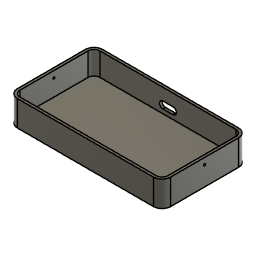
Case (INCOMPLETE) (Autodesk Fusion 360 design; units mm, degrees)
Autodesk Fusion 360 part; units mm, degrees
sketch "Sketch1" plane through (0, 0, 0) normal (0, 1, 0) x (1, 0, 0)
  line L0 (-80, 50) -> (80, 50)
  line L1 (90, 40) -> (90, -40)
  line L2 (80, -50) -> (-80, -50)
  line L3 (-90, -40) -> (-90, 40)
  line L4 (-90, 50) -> (90, -50) construction
  line L5 (90, 50) -> (-90, -50) construction
  arc A0 (-90, -40) -> (-80, -50) centre (-80, -40) ccw
  arc A1 (80, -50) -> (90, -40) centre (80, -40) ccw
  arc A2 (90, 40) -> (80, 50) centre (80, 40) ccw
  arc A3 (-80, 50) -> (-90, 40) centre (-80, 40) ccw
  arc A4 (87, 40) -> (80, 47) centre (80, 40) ccw
  line L6 (-80, 47) -> (80, 47)
  arc A5 (-80, 47) -> (-87, 40) centre (-80, 40) ccw
  line L7 (-87, -40) -> (-87, 40)
  arc A6 (-87, -40) -> (-80, -47) centre (-80, -40) ccw
  line L8 (80, -47) -> (-80, -47)
  arc A7 (80, -47) -> (87, -40) centre (80, -40) ccw
  line L9 (87, 40) -> (87, -40)
  dimension "d1" = 180
  dimension "d2" = 100
  dimension "d3" = 10
  dimension "d4" = 3
  constraint horizontal L0
  constraint perpendicular L0 L1
  constraint parallel L0 L2
  constraint parallel L1 L3
  constraint coincident L4 origin
  constraint coincident L5 origin
  constraint coincident L5.end L3
  constraint coincident L5.end L2
  constraint tangent L3 A0
  constraint tangent L2 A0
  constraint coincident L4.end L2
  constraint coincident L4.end L1
  constraint tangent L2 A1
  constraint tangent L1 A1
  constraint equal A0 A1
  constraint coincident L5.start L1
  constraint coincident L5.start L0
  constraint tangent L1 A2
  constraint tangent L0 A2
  constraint equal A0 A2
  constraint coincident L4.start L0
  constraint coincident L4.start L3
  constraint tangent L0 A3
  constraint tangent L3 A3
  constraint equal A0 A3
  measures "d1" distance of L4.end L5.end
  measures "d2" distance of L5.start L4.end
  measures "d3" radius of A0
extrude "Extrude1" add sketch "Sketch1" along normal blind 3 contours L0 L1 L2 L3 A0 A1 A2 A3 | A4 L6 A5 L7 A6 L8 A7 L9
extrude "Extrude2" cut sketch "Sketch1" along normal blind 25
extrude "Extrude3" add sketch "Sketch1" along normal blind 30
sketch "Sketch2" plane through (0, 0, -50) normal (0, 0, -1) x (-1, 0, 0)
  line L0 (-80, 0) -> (80, 0)
  line L1 (80, 0) -> (80, 30)
  line L2 (80, 30) -> (-80, 30)
  line L3 (-80, 30) -> (-80, 0)
  line L4 (6, 16) -> (-6, 16)
  arc A0 (-6, 16) -> (-6, 8) centre (-6, 12) ccw
  line L5 (-6, 8) -> (6, 8)
  arc A1 (6, 8) -> (6, 16) centre (6, 12) ccw
  line L6 (6, 12) -> (-6, 12) construction
  line L7 (80, 0) -> (-80, 0)
  dimension "d11" = 12
  dimension "d12" = 8
  dimension "d13" = 8
  dimension "d25" = 6
  constraint tangent L4 A0
  constraint tangent A0 L5
  constraint parallel L4 L5
  constraint tangent L5 A1
  constraint tangent L4 A1
  constraint horizontal L6
  measures "d11" distance of A1.centre A0.centre
  measures "d12" diameter of A0
  measures "d13" distance of L5 L7
  measures "d25" horizontal distance of origin A0.end
extrude "Extrude4" cut sketch "Sketch2" against normal blind 3 contours L4 A0 L5 A1
sketch "Sketch5" plane through (90, 0, 0) normal (1, 0, 0) x (0, 0, -1)
  line L0 (-40, 0) -> (40, 0)
  line L1 (40, 0) -> (40, 30)
  line L2 (40, 30) -> (-40, 30)
  line L3 (-40, 30) -> (-40, 0)
  circle A0 centre (0, 22.5) radius 1.25
  dimension "d21" = 2.5
  dimension "d22" = 7.5
  measures "d21" diameter of A0
  measures "d22" distance of L2 A0.centre
extrude "Extrude6" cut sketch "Sketch5" against normal blind 32423432 contours A0
sketch "Sketch4" plane through (100, 0, 0) normal (1, 0, 0) x (0, 0, -1)
  line L0 (-50, 0) -> (50, 0)
  line L1 (50, 0) -> (50, 30)
  line L2 (50, 30) -> (-50, 30)
  line L3 (-50, 30) -> (-50, 0)
  circle A0 centre (0, 22.5) radius 1
  dimension "d17" = 2
  dimension "d18" = 7.5
  measures "d17" diameter of A0
  measures "d18" distance of L2 A0.centre
extrude "Extrude5" cut sketch "Sketch4" against normal blind 23434 contours A0
equation "d13 = 3 mm + 5 mm"
equation "d18 = ( 15 / 2 ) * 1 mm"
equation "d22 = ( 15 / 2 ) * 1 mm"
equation "d25 = ( 12 / 2 ) * 1 mm"
